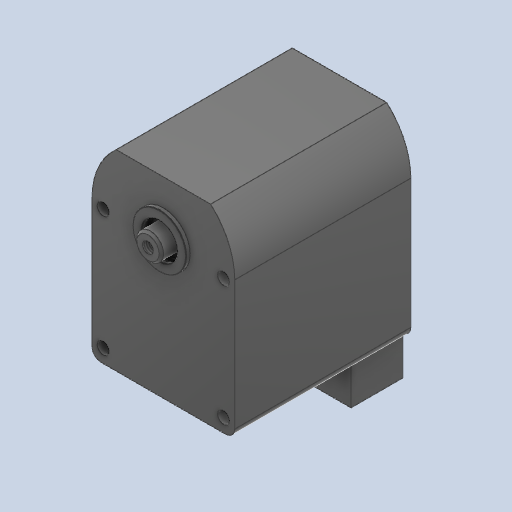
# Autodesk Inventor part: B3M-SC-1170-A
Saved by Autodesk Inventor 2022 (Build 260153000, 153)
## iProperties
Part Number: B3M-SC-1170-A
Material: 一般
Document SubType Name: Modeling
Designer: Masato Kubotera
Density: 1 g/cm^3
Appearance: 滑らか - 黒
Mass: 54.9026 g
Surface Area: 108.76 cm^2
Volume: 54.9026 cm^3
Description: ReadyMade
Catalog Web Link: https://kondo-robot.com/product/03092
Author: Masato Kubotera
Autodesk Inventor part; units mm, degrees
ref_plane "YZ Plane" through (0, 0, 0) normal (1, 0, 0) x (0, 1, 0)
ref_plane "XZ Plane" through (0, 0, 0) normal (0, 1, 0) x (-1, 0, 0)
ref_plane "XY Plane" through (0, 0, 0) normal (0, 0, 1) x (1, 0, 0)
sketch "スケッチ1" plane through (0, 0, 0) normal (0, 0, 1) x (1, 0, 0)
  line L0 (-16, 21.5) -> (-10.583, 21.5) construction
  line L1 (16, 21.5) -> (16, 9.5) construction
  line L2 (16, -21.5) -> (-16, -21.5)
  line L3 (-16, -21.5) -> (-16, 9.5)
  line L4 (-16, 21.5) -> (16, -21.5) construction
  line L5 (16, 21.5) -> (-16, -21.5) construction
  line L6 (-14.4, -21.5) -> (-14.4, -30)
  line L7 (-14.4, -30) -> (14.4, -30)
  line L8 (0, 21.5) -> (0, -21.5) construction
  line L9 (14.4, -21.5) -> (14.4, -30)
  line L10 (-13.5, 21.5) -> (-13.5, -21.5) construction
  circle A0 centre (0, 9.5) radius 6
  circle A1 centre (0, 9.5) radius 4
  arc A2 (-10.583, 21.5) -> (-16, 9.5) centre (0, 9.5) ccw
  arc A3 (16, 9.5) -> (10.583, 21.5) centre (0, 9.5) ccw
  line L11 (-10.583, 21.5) -> (10.583, 21.5)
  line L12 (-16, 9.5) -> (-16, 21.5) construction
  line L13 (10.583, 21.5) -> (16, 21.5) construction
  line L14 (16, 9.5) -> (16, -21.5)
  circle A4 centre (0, 9.5) radius 3
  circle A5 centre (0, 9.5) radius 4.8
  point P0 (0, 0)
  point P1 (-13.5, 8.5)
  point P2 (-13.5, -18.5)
  point P3 (13.5, 8.5)
  point P4 (13.5, -18.5)
  dimension "d0" = 32
  dimension "d1" = 43
  dimension "d4" = 28.8
  dimension "d5" = 8.5
  dimension "d8" = 27
  dimension "d9" = 8.5
  dimension "d12" = 18.5
  dimension "d13" = 12
  dimension "d14" = 8
  dimension "d15" = 9.5
  dimension "d17" = 16
  dimension "d32" = 13.5
  dimension "d47" = 6
  dimension "d67" = 9.6
  constraints: 30 end point, 8 perpendicular, 7 parallel, 6 centre point, 6 point on line, 6 symmetric about line, 4 coincident, 4 midpoint, 4 point on circle, 3 horizontal, 1 vertical, 1 other
  measures "d0" distance of L2.start L2.end
  measures "d1" distance of L1.start L2.start
  measures "d4" distance of L6.end L7.end
  measures "d5" distance of L7.end L9.start
  measures "d8" distance of point (-13.5, -18.5) point (-13.5, 8.5)
  measures "d9" vertical distance of point (-13.5, 8.5) point (0, 0)
  measures "d12" vertical distance of point (-13.5, -18.5) point (0, 0)
  measures "d13" diameter of A0
  measures "d14" diameter of A1
  measures "d15" distance of point (0, 0) A0.centre
  measures "d17" radius of A2
  measures "d32" horizontal distance of L10.start point (0, 0)
  measures "d47" diameter of A4
  measures "d67" diameter of A5
extrude "押し出し1" add sketch "スケッチ1" against normal blind 12.2 contours L2 L3 A2 L11 A3 L14 | A0 | A1 | A4 | A5
extrude "押し出し2" add sketch "スケッチ1" against normal blind 12 contours L9 L7 L6 L2
extrude "押し出し3" add sketch "スケッチ1" against normal blind 14 contours A0 | A1 | A4 | A5
extrude "押し出し4" add sketch "スケッチ1" against normal blind 17.7 contours A1 | A4
chamfer "面取り1" distance 1.2 angle 45 1 edges at (-6, 9.5, -14)
sketch "スケッチ2" plane through (0, 9.5, -17.7) normal (0, 0, -1) x (-1, 0, 0)
  circle A0 centre (0, 0) radius 4 projected
  point P0 (0, -9.5)
  constraints: 1 coincident
hole "穴1" at (0, 9.5, -17.7) direction (0, 0, 1) diameter 2.459 depth 6 thread size "M3x0.5" class "6H" standard "ANSI Metric M Profile"
extrude "押し出し5" add sketch "スケッチ1" along normal blind 27.3 contours L2 L3 A2 L11 A3 L14 | A0 | A1 | A4 | A5
hole "穴2" at (-13.5, 8.5, 0) at (-13.5, -18.5, 0) at (13.5, 8.5, 0) at (13.5, -18.5, 0) direction (0, 0, 1) diameter 2.7 end through all both
extrude "押し出し6" cut sketch "スケッチ1" against normal blind 0.4 contours L9 L7 L6 L2
fillet "フィレット1" radius 2 2 edges at (16, -21.5, 7.55) (-16, -21.5, 7.55)
extrude "押し出し7" add sketch "スケッチ1" along normal blind 28.2 contours A0 | A1 | A4 | A5
extrude "押し出し8" add sketch "スケッチ1" along normal blind 30.75 contours A4
sketch "スケッチ3" plane through (0, 9.5, 30.75) normal (0, 0, 1) x (1, 0, 0)
  circle A0 centre (0, 0) radius 1.2295 projected
  point P0 (0, -9.5)
  constraints: 1 coincident
hole "穴3" at (0, 9.5, 30.75) direction (0, 0, -1) diameter 2.459 end through all thread size "M3x0.5" class "6H" standard "ANSI Metric M Profile"
sketch "スケッチ4" plane through (0, 9.5, 28.2) normal (0, 0, 1) x (1, 0, 0)
  circle A0 centre (0, 0) radius 4
  circle A1 centre (0, 0) radius 3
  point P0 (0, -9.5)
  constraints: 2 centre point, 1 coincident
extrude "押し出し9" cut sketch "スケッチ4" against normal blind 2.3
chamfer "面取り2" distance 0.5 angle 45 1 edges at (-3, 9.5, 30.75)
extrude "押し出し10" add sketch "スケッチ1" against normal blind 14.2 contours A5
chamfer "面取り4" distance 0.1 angle 45 2 edges at (-6, 9.5, 28.2) (-4, 9.5, 28.2)
